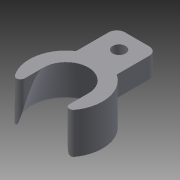
# Autodesk Inventor part: brush rack
Saved by Autodesk Inventor 2013 SP2 (Build 170200200, 200)
## iProperties
Created: 2017-05-15
Part Number: brush rack
Material: Generic
Document SubType Name: Modeling
Designer: Herman de Vries
Density: 1 g/cm^3
Author: Herman de Vries
Autodesk Inventor part; units mm, degrees
ref_plane "YZ Plane" through (0, 0, 0) normal (1, 0, 0) x (0, 1, 0)
ref_plane "XZ Plane" through (0, 0, 0) normal (0, 1, 0) x (-1, 0, 0)
ref_plane "XY Plane" through (0, 0, 0) normal (0, 0, 1) x (1, 0, 0)
sketch "Sketch1" plane through (0, 0, 0) normal (1, 0, 0) x (0, 1, 0)
  line L0 (5.5, 10) -> (5.5, 10)
  line L1 (8.5, 0) -> (9, 0)
  line L2 (9, 0) -> (9, 10)
  line L3 (9, 10) -> (5.5, 10)
  line L4 (0, 0) -> (0, 4.238)
  line L5 (5.5, 10) -> (8.5, 0)
  dimension "d11" = 0
  dimension "d13" = 9
  dimension "d14" = 5.5
  dimension "d15" = 10
  dimension "d26" = 8.5
  constraints: 12 end point, 2 horizontal, 1 horizontal alignment, 1 perpendicular, 1 vertical
  measures "d11" distance of L0.start L0.end
  measures "d13" distance from line of L4.start L2
  measures "d14" horizontal distance of L4.start L0.start
  measures "d15" distance of L1.end L2.end
  measures "d26" distance of L1.start L4.start
revolve "Revolution1" add sketch "Sketch1" angle 360 about axis through (0, 0, 0) along (0, 0, 1)
sketch "Sketch3" plane through (0, 0, 0) normal (0, 0, -1) x (-1, 0, 0)
  line L0 (-5.5, 0) -> (5.5, 0)
  line L1 (5.5, 0) -> (5.5, -9)
  line L2 (5.5, -9) -> (-5.5, -9)
  line L3 (-5.5, -9) -> (-5.5, 0)
  circle A0 centre (0, 0) radius 9 projected
  circle A1 centre (0, 0) radius 5.5 projected
  constraints: 8 end point, 2 parallel, 2 point on circle, 1 horizontal, 1 perpendicular, 1 tangent
extrude "Extrusion1" cut sketch "Sketch3" against normal blind 10 contours A1 L1 A0 L3 | L0 A1 | A0 L2 L3 | L1 L2 A0 picked at (4.148, -6.5999) picked at (-1.2514, -2.3608)
fillet "Fillet1" radius 1 5 edges at (0, 8.5, 0) (5.5, -6.8023, 0) (-5.5, -6.8023, 0) (-5.5, -7.1239, 5) (5.5, -7.1239, 5)
sketch "Sketch4" plane through (0, 0, 10) normal (0, 0, 1) x (1, 0, 0)
  line L0 (-5, 17.4833) -> (5, 17.4833)
  line L1 (5, 17.4833) -> (5, 7.4833)
  line L2 (5, 7.4833) -> (-5, 7.4833)
  line L3 (-5, 7.4833) -> (-5, 17.4833)
  circle A0 centre (0, 13.0699) radius 1.6
  arc A1 (7.3125, -5.2467) -> (-7.3125, -5.2467) centre (0, 0) ccw projected
  dimension "d19" = 10
  dimension "d21" = 10
  dimension "d22" = 3.2
  dimension "d29" = 4.4135
  constraints: 8 end point, 2 parallel, 2 point on circle, 1 centre point, 1 horizontal, 1 perpendicular
  measures "d19" distance of L0.start L0.end
  measures "d21" distance of L2.end L0.start
  measures "d22" diameter of A0
  measures "d29" distance from line of A0.centre L0
extrude "Extrusion2" add sketch "Sketch4" against normal blind 5 contours L0 L1 A1 L3
fillet "Fillet2" radius 2 2 edges at (5, 17.4833, 7.5) (-5, 17.4833, 7.5)
body "Solid1"
